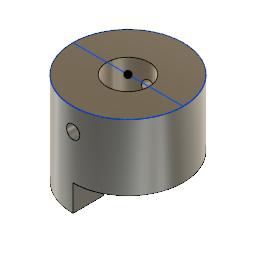
Rotational Link v1 (Autodesk Fusion 360 design; units mm, degrees)
Autodesk Fusion 360 part; units mm, degrees
mesh "Mesh1" [no effect]
sketch "Sketch1" plane through (0, 0, 0) normal (0, 0, 1) x (1, 0, 0)
  spline S0 degree 5 poles (-0.6, 6.1514) (-0.576, 6.0983) (-0.528, 5.9968) (-0.456, 5.8583) (-0.36, 5.7021) (-0.24, 5.5571) (-0.12, 5.4669) (0, 5.436) (0.12, 5.4669) (0.24, 5.5571) (0.36, 5.7021) (0.456, 5.8583) (0.528, 5.9968) (0.576, 6.0983) (0.6, 6.1514) knots 0 0 0 0 0 0 0.1 0.2 0.3 0.4 0.5 0.6 0.7 0.8 0.9 1 1 1 1 1 1
  spline S1 degree 5 poles (-0.6, 6.1514) (-0.576, 6.0983) (-0.528, 5.9968) (-0.456, 5.8583) (-0.36, 5.7021) (-0.24, 5.5571) (-0.12, 5.4669) (0, 5.436) (0.12, 5.4669) (0.24, 5.5571) (0.36, 5.7021) (0.456, 5.8583) (0.528, 5.9968) (0.576, 6.0983) (0.6, 6.1514) knots 0 0 0 0 0 0 0.1 0.2 0.3 0.4 0.5 0.6 0.7 0.8 0.9 1 1 1 1 1 1
  line L0 (0.6, 6.1514) -> (1.3338, 6.0301)
  spline S2 degree 5 poles (-2.4715, 5.6649) (-2.4323, 5.6218) (-2.3553, 5.5401) (-2.244, 5.4307) (-2.1044, 5.3117) (-1.9455, 5.2109) (-1.8035, 5.1622) (-1.6798, 5.1699) (-1.5752, 5.2364) (-1.489, 5.3592) (-1.4197, 5.5342) (-1.3767, 5.7125) (-1.3509, 5.8664) (-1.3367, 5.9778) (-1.3303, 6.0357) knots 0 0 0 0 0 0 0.1 0.2 0.3 0.4 0.5 0.6 0.7 0.8 0.9 1 1 1 1 1 1
  line L1 (-1.3303, 6.0357) -> (-0.5949, 6.1471)
  spline S3 degree 5 poles (-4.1011, 4.6239) (-4.0505, 4.5951) (-3.952, 4.5411) (-3.8124, 4.4715) (-3.6428, 4.4015) (-3.4605, 4.3547) (-3.3104, 4.3523) (-3.1952, 4.3978) (-3.1163, 4.4933) (-3.0722, 4.6368) (-3.0603, 4.8247) (-3.0745, 5.0075) (-3.0976, 5.1618) (-3.1185, 5.2722) (-3.1303, 5.3292) knots 0 0 0 0 0 0 0.1 0.2 0.3 0.4 0.5 0.6 0.7 0.8 0.9 1 1 1 1 1 1
  line L2 (-3.1303, 5.3292) -> (-2.4653, 5.6624)
  spline S4 degree 5 poles (-5.3293, 3.1303) (-5.2722, 3.1185) (-5.1618, 3.0976) (-5.0075, 3.0745) (-4.8247, 3.0603) (-4.6368, 3.0722) (-4.4933, 3.1163) (-4.3978, 3.1952) (-4.3523, 3.3104) (-4.3547, 3.4605) (-4.4015, 3.6428) (-4.4715, 3.8123) (-4.5411, 3.952) (-4.5951, 4.0505) (-4.6239, 4.1011) knots 0 0 0 0 0 0 0.1 0.2 0.3 0.4 0.5 0.6 0.7 0.8 0.9 1 1 1 1 1 1
  line L3 (-4.6239, 4.1011) -> (-4.0944, 4.6234)
  spline S5 degree 5 poles (-6.0357, 1.3302) (-5.9778, 1.3367) (-5.8664, 1.3509) (-5.7125, 1.3766) (-5.5342, 1.4196) (-5.3592, 1.489) (-5.2364, 1.5752) (-5.1699, 1.6798) (-5.1622, 1.8035) (-5.2109, 1.9455) (-5.3117, 2.1044) (-5.4307, 2.244) (-5.5401, 2.3552) (-5.6218, 2.4323) (-5.6649, 2.4715) knots 0 0 0 0 0 0 0.1 0.2 0.3 0.4 0.5 0.6 0.7 0.8 0.9 1 1 1 1 1 1
  line L4 (-5.6649, 2.4715) -> (-5.3228, 3.1319)
  spline S6 degree 5 poles (-6.1514, -0.6) (-6.0983, -0.576) (-5.9968, -0.528) (-5.8583, -0.456) (-5.7021, -0.36) (-5.5571, -0.24) (-5.4669, -0.12) (-5.436, 0) (-5.4669, 0.12) (-5.5571, 0.24) (-5.7021, 0.36) (-5.8583, 0.456) (-5.9968, 0.528) (-6.0983, 0.576) (-6.1514, 0.6) knots 0 0 0 0 0 0 0.1 0.2 0.3 0.4 0.5 0.6 0.7 0.8 0.9 1 1 1 1 1 1
  line L5 (-6.1514, 0.6) -> (-6.0301, 1.3338)
  spline S7 degree 5 poles (-5.6649, -2.4715) (-5.6218, -2.4323) (-5.5401, -2.3553) (-5.4307, -2.244) (-5.3117, -2.1044) (-5.2109, -1.9455) (-5.1622, -1.8035) (-5.1699, -1.6798) (-5.2364, -1.5752) (-5.3592, -1.489) (-5.5342, -1.4197) (-5.7125, -1.3767) (-5.8664, -1.3509) (-5.9778, -1.3367) (-6.0357, -1.3303) knots 0 0 0 0 0 0 0.1 0.2 0.3 0.4 0.5 0.6 0.7 0.8 0.9 1 1 1 1 1 1
  line L6 (-6.0357, -1.3303) -> (-6.1471, -0.5949)
  spline S8 degree 5 poles (-4.6239, -4.1011) (-4.5951, -4.0505) (-4.5411, -3.952) (-4.4715, -3.8124) (-4.4015, -3.6428) (-4.3547, -3.4605) (-4.3523, -3.3104) (-4.3978, -3.1952) (-4.4933, -3.1163) (-4.6368, -3.0722) (-4.8247, -3.0603) (-5.0075, -3.0745) (-5.1618, -3.0976) (-5.2722, -3.1185) (-5.3292, -3.1303) knots 0 0 0 0 0 0 0.1 0.2 0.3 0.4 0.5 0.6 0.7 0.8 0.9 1 1 1 1 1 1
  line L7 (-5.3292, -3.1303) -> (-5.6624, -2.4653)
  spline S9 degree 5 poles (-3.1303, -5.3293) (-3.1185, -5.2722) (-3.0976, -5.1618) (-3.0745, -5.0075) (-3.0603, -4.8247) (-3.0722, -4.6368) (-3.1163, -4.4933) (-3.1952, -4.3978) (-3.3104, -4.3523) (-3.4605, -4.3547) (-3.6428, -4.4015) (-3.8123, -4.4715) (-3.952, -4.5411) (-4.0505, -4.5951) (-4.1011, -4.6239) knots 0 0 0 0 0 0 0.1 0.2 0.3 0.4 0.5 0.6 0.7 0.8 0.9 1 1 1 1 1 1
  line L8 (-4.1011, -4.6239) -> (-4.6234, -4.0944)
  spline S10 degree 5 poles (-1.3302, -6.0357) (-1.3367, -5.9778) (-1.3509, -5.8664) (-1.3766, -5.7125) (-1.4196, -5.5342) (-1.489, -5.3592) (-1.5752, -5.2364) (-1.6798, -5.1699) (-1.8035, -5.1622) (-1.9455, -5.2109) (-2.1044, -5.3117) (-2.244, -5.4307) (-2.3552, -5.5401) (-2.4323, -5.6218) (-2.4715, -5.6649) knots 0 0 0 0 0 0 0.1 0.2 0.3 0.4 0.5 0.6 0.7 0.8 0.9 1 1 1 1 1 1
  line L9 (-2.4715, -5.6649) -> (-3.1319, -5.3228)
  spline S11 degree 5 poles (0.6, -6.1514) (0.576, -6.0983) (0.528, -5.9968) (0.456, -5.8583) (0.36, -5.7021) (0.24, -5.5571) (0.12, -5.4669) (0, -5.436) (-0.12, -5.4669) (-0.24, -5.5571) (-0.36, -5.7021) (-0.456, -5.8583) (-0.528, -5.9968) (-0.576, -6.0983) (-0.6, -6.1514) knots 0 0 0 0 0 0 0.1 0.2 0.3 0.4 0.5 0.6 0.7 0.8 0.9 1 1 1 1 1 1
  line L10 (-0.6, -6.1514) -> (-1.3338, -6.0301)
  spline S12 degree 5 poles (2.4715, -5.6649) (2.4323, -5.6218) (2.3553, -5.5401) (2.244, -5.4307) (2.1044, -5.3117) (1.9455, -5.2109) (1.8035, -5.1622) (1.6798, -5.1699) (1.5752, -5.2364) (1.489, -5.3592) (1.4197, -5.5342) (1.3767, -5.7125) (1.3509, -5.8664) (1.3367, -5.9778) (1.3303, -6.0357) knots 0 0 0 0 0 0 0.1 0.2 0.3 0.4 0.5 0.6 0.7 0.8 0.9 1 1 1 1 1 1
  line L11 (1.3303, -6.0357) -> (0.5949, -6.1471)
  spline S13 degree 5 poles (4.1011, -4.6239) (4.0505, -4.5951) (3.952, -4.5411) (3.8124, -4.4715) (3.6428, -4.4015) (3.4605, -4.3547) (3.3104, -4.3523) (3.1952, -4.3978) (3.1163, -4.4933) (3.0722, -4.6368) (3.0603, -4.8247) (3.0745, -5.0075) (3.0976, -5.1618) (3.1185, -5.2722) (3.1303, -5.3292) knots 0 0 0 0 0 0 0.1 0.2 0.3 0.4 0.5 0.6 0.7 0.8 0.9 1 1 1 1 1 1
  line L12 (3.1303, -5.3292) -> (2.4653, -5.6624)
  spline S14 degree 5 poles (5.3293, -3.1303) (5.2722, -3.1185) (5.1618, -3.0976) (5.0075, -3.0745) (4.8247, -3.0603) (4.6368, -3.0722) (4.4933, -3.1163) (4.3978, -3.1952) (4.3523, -3.3104) (4.3547, -3.4605) (4.4015, -3.6428) (4.4715, -3.8123) (4.5411, -3.952) (4.5951, -4.0505) (4.6239, -4.1011) knots 0 0 0 0 0 0 0.1 0.2 0.3 0.4 0.5 0.6 0.7 0.8 0.9 1 1 1 1 1 1
  line L13 (4.6239, -4.1011) -> (4.0944, -4.6234)
  spline S15 degree 5 poles (6.0357, -1.3302) (5.9778, -1.3367) (5.8664, -1.3509) (5.7125, -1.3766) (5.5342, -1.4196) (5.3592, -1.489) (5.2364, -1.5752) (5.1699, -1.6798) (5.1622, -1.8035) (5.2109, -1.9455) (5.3117, -2.1044) (5.4307, -2.244) (5.5401, -2.3552) (5.6218, -2.4323) (5.6649, -2.4715) knots 0 0 0 0 0 0 0.1 0.2 0.3 0.4 0.5 0.6 0.7 0.8 0.9 1 1 1 1 1 1
  line L14 (5.6649, -2.4715) -> (5.3228, -3.1319)
  spline S16 degree 5 poles (6.1514, 0.6) (6.0983, 0.576) (5.9968, 0.528) (5.8583, 0.456) (5.7021, 0.36) (5.5571, 0.24) (5.4669, 0.12) (5.436, 0) (5.4669, -0.12) (5.5571, -0.24) (5.7021, -0.36) (5.8583, -0.456) (5.9968, -0.528) (6.0983, -0.576) (6.1514, -0.6) knots 0 0 0 0 0 0 0.1 0.2 0.3 0.4 0.5 0.6 0.7 0.8 0.9 1 1 1 1 1 1
  line L15 (6.1514, -0.6) -> (6.0301, -1.3338)
  spline S17 degree 5 poles (5.6649, 2.4715) (5.6218, 2.4323) (5.5401, 2.3553) (5.4307, 2.244) (5.3117, 2.1044) (5.2109, 1.9455) (5.1622, 1.8035) (5.1699, 1.6798) (5.2364, 1.5752) (5.3592, 1.489) (5.5342, 1.4197) (5.7125, 1.3767) (5.8664, 1.3509) (5.9778, 1.3367) (6.0357, 1.3303) knots 0 0 0 0 0 0 0.1 0.2 0.3 0.4 0.5 0.6 0.7 0.8 0.9 1 1 1 1 1 1
  line L16 (6.0357, 1.3303) -> (6.1471, 0.5949)
  spline S18 degree 5 poles (4.6239, 4.1011) (4.5951, 4.0505) (4.5411, 3.952) (4.4715, 3.8124) (4.4015, 3.6428) (4.3547, 3.4605) (4.3523, 3.3104) (4.3978, 3.1952) (4.4933, 3.1163) (4.6368, 3.0722) (4.8247, 3.0603) (5.0075, 3.0745) (5.1618, 3.0976) (5.2722, 3.1185) (5.3292, 3.1303) knots 0 0 0 0 0 0 0.1 0.2 0.3 0.4 0.5 0.6 0.7 0.8 0.9 1 1 1 1 1 1
  line L17 (5.3292, 3.1303) -> (5.6624, 2.4653)
  spline S19 degree 5 poles (3.1303, 5.3293) (3.1185, 5.2722) (3.0976, 5.1618) (3.0745, 5.0075) (3.0603, 4.8247) (3.0722, 4.6368) (3.1163, 4.4933) (3.1952, 4.3978) (3.3104, 4.3523) (3.4605, 4.3547) (3.6428, 4.4015) (3.8123, 4.4715) (3.952, 4.5411) (4.0505, 4.5951) (4.1011, 4.6239) knots 0 0 0 0 0 0 0.1 0.2 0.3 0.4 0.5 0.6 0.7 0.8 0.9 1 1 1 1 1 1
  line L18 (4.1011, 4.6239) -> (4.6234, 4.0944)
  spline S20 degree 5 poles (1.3302, 6.0357) (1.3367, 5.9778) (1.3509, 5.8664) (1.3766, 5.7125) (1.4196, 5.5342) (1.489, 5.3592) (1.5752, 5.2364) (1.6798, 5.1699) (1.8035, 5.1622) (1.9455, 5.2109) (2.1044, 5.3117) (2.244, 5.4307) (2.3552, 5.5401) (2.4323, 5.6218) (2.4715, 5.6649) knots 0 0 0 0 0 0 0.1 0.2 0.3 0.4 0.5 0.6 0.7 0.8 0.9 1 1 1 1 1 1
  line L19 (2.4715, 5.6649) -> (3.1319, 5.3228)
  circle A0 centre (0, 0) radius 12.5
  point P0 (0, 5.4514)
  point P1 (0, 5.4514)
  point P2 (-1.6846, 5.1846)
  point P3 (-3.2043, 4.4103)
  point P4 (-4.4103, 3.2042)
  point P5 (-5.1846, 1.6846)
  point P6 (-5.4514, 0)
  point P7 (-5.1846, -1.6846)
  point P8 (-4.4103, -3.2043)
  point P9 (-3.2042, -4.4103)
  point P10 (-1.6846, -5.1846)
  point P11 (0, -5.4514)
  point P12 (1.6846, -5.1846)
  point P13 (3.2043, -4.4103)
  point P14 (4.4103, -3.2042)
  point P15 (5.1846, -1.6846)
  point P16 (5.4514, 0)
  point P17 (5.1846, 1.6846)
  point P18 (4.4103, 3.2043)
  point P19 (3.2042, 4.4103)
  point P20 (1.6846, 5.1846)
  constraint coincident A0.centre origin
extrude "Extrude1" add sketch "Sketch1" along normal blind 6
sketch "Sketch2" plane through (0, 0, 6) normal (0, 0, 1) x (-1, 0, 0)
  spline S0 degree 5 poles (-1.3308, -6.0305) (-1.3372, -5.9738) (-1.3514, -5.8637) (-1.377, -5.7109) (-1.4199, -5.5336) (-1.489, -5.3592) (-1.5752, -5.2364) (-1.6798, -5.1699) (-1.8035, -5.1622) (-1.9455, -5.2109) (-2.1044, -5.3117) (-2.244, -5.4307) (-2.3552, -5.5401) (-2.4323, -5.6218) (-2.4715, -5.6649) knots 0.001796 0.001796 0.001796 0.001796 0.001796 0.001796 0.1 0.2 0.3 0.4 0.5 0.6 0.7 0.8 0.9 1 1 1 1 1 1
  line L0 (-2.4715, -5.6649) -> (-3.1292, -5.3241)
  spline S1 degree 5 poles (-3.1292, -5.3241) (-3.1177, -5.2682) (-3.0972, -5.1591) (-3.0744, -5.0059) (-3.0604, -4.824) (-3.0722, -4.6368) (-3.1163, -4.4933) (-3.1952, -4.3978) (-3.3104, -4.3523) (-3.4605, -4.3547) (-3.6428, -4.4015) (-3.8123, -4.4715) (-3.952, -4.5411) (-4.0505, -4.5951) (-4.1011, -4.6239) knots 0.001796 0.001796 0.001796 0.001796 0.001796 0.001796 0.1 0.2 0.3 0.4 0.5 0.6 0.7 0.8 0.9 1 1 1 1 1 1
  line L1 (-4.1011, -4.6239) -> (-4.6213, -4.0966)
  spline S2 degree 5 poles (-4.6213, -4.0966) (-4.5931, -4.047) (-4.5399, -3.9495) (-4.4708, -3.8108) (-4.4013, -3.6422) (-4.3547, -3.4605) (-4.3523, -3.3104) (-4.3978, -3.1952) (-4.4933, -3.1163) (-4.6368, -3.0722) (-4.8247, -3.0603) (-5.0075, -3.0745) (-5.1618, -3.0976) (-5.2722, -3.1185) (-5.3292, -3.1303) knots 0.001796 0.001796 0.001796 0.001796 0.001796 0.001796 0.1 0.2 0.3 0.4 0.5 0.6 0.7 0.8 0.9 1 1 1 1 1 1
  line L2 (-5.3292, -3.1303) -> (-5.6611, -2.468)
  spline S3 degree 5 poles (-5.6611, -2.468) (-5.6189, -2.4295) (-5.5381, -2.3533) (-5.4296, -2.2428) (-5.3114, -2.1039) (-5.2109, -1.9455) (-5.1622, -1.8035) (-5.1699, -1.6798) (-5.2364, -1.5752) (-5.3592, -1.489) (-5.5342, -1.4197) (-5.7125, -1.3767) (-5.8664, -1.3509) (-5.9778, -1.3367) (-6.0357, -1.3303) knots 0.001796 0.001796 0.001796 0.001796 0.001796 0.001796 0.1 0.2 0.3 0.4 0.5 0.6 0.7 0.8 0.9 1 1 1 1 1 1
  line L3 (-6.0357, -1.3303) -> (-6.1466, -0.5979)
  spline S4 degree 5 poles (-6.1466, -0.5979) (-6.0947, -0.5743) (-5.9943, -0.5267) (-5.8569, -0.4551) (-5.7015, -0.3596) (-5.5571, -0.24) (-5.4669, -0.12) (-5.436, 0) (-5.4669, 0.12) (-5.5571, 0.24) (-5.7021, 0.36) (-5.8583, 0.456) (-5.9968, 0.528) (-6.0983, 0.576) (-6.1514, 0.6) knots 0.001796 0.001796 0.001796 0.001796 0.001796 0.001796 0.1 0.2 0.3 0.4 0.5 0.6 0.7 0.8 0.9 1 1 1 1 1 1
  line L4 (-6.1514, 0.6) -> (-6.0305, 1.3308)
  spline S5 degree 5 poles (-6.0305, 1.3308) (-5.9738, 1.3372) (-5.8637, 1.3514) (-5.7109, 1.377) (-5.5336, 1.4199) (-5.3592, 1.489) (-5.2364, 1.5752) (-5.1699, 1.6798) (-5.1622, 1.8035) (-5.2109, 1.9455) (-5.3117, 2.1044) (-5.4307, 2.244) (-5.5401, 2.3552) (-5.6218, 2.4323) (-5.6649, 2.4715) knots 0.001796 0.001796 0.001796 0.001796 0.001796 0.001796 0.1 0.2 0.3 0.4 0.5 0.6 0.7 0.8 0.9 1 1 1 1 1 1
  line L5 (-5.6649, 2.4715) -> (-5.3241, 3.1292)
  spline S6 degree 5 poles (-5.3241, 3.1292) (-5.2682, 3.1177) (-5.1591, 3.0972) (-5.0059, 3.0744) (-4.824, 3.0604) (-4.6368, 3.0722) (-4.4933, 3.1163) (-4.3978, 3.1952) (-4.3523, 3.3104) (-4.3547, 3.4605) (-4.4015, 3.6428) (-4.4715, 3.8123) (-4.5411, 3.952) (-4.5951, 4.0505) (-4.6239, 4.1011) knots 0.001796 0.001796 0.001796 0.001796 0.001796 0.001796 0.1 0.2 0.3 0.4 0.5 0.6 0.7 0.8 0.9 1 1 1 1 1 1
  line L6 (-4.6239, 4.1011) -> (-4.0966, 4.6213)
  spline S7 degree 5 poles (-4.0966, 4.6213) (-4.047, 4.5931) (-3.9495, 4.5399) (-3.8108, 4.4708) (-3.6422, 4.4013) (-3.4605, 4.3547) (-3.3104, 4.3523) (-3.1952, 4.3978) (-3.1163, 4.4933) (-3.0722, 4.6368) (-3.0603, 4.8247) (-3.0745, 5.0075) (-3.0976, 5.1618) (-3.1185, 5.2722) (-3.1303, 5.3292) knots 0.001796 0.001796 0.001796 0.001796 0.001796 0.001796 0.1 0.2 0.3 0.4 0.5 0.6 0.7 0.8 0.9 1 1 1 1 1 1
  line L7 (-3.1303, 5.3292) -> (-2.468, 5.6611)
  spline S8 degree 5 poles (-2.468, 5.6611) (-2.4295, 5.6189) (-2.3533, 5.5381) (-2.2428, 5.4296) (-2.1039, 5.3114) (-1.9455, 5.2109) (-1.8035, 5.1622) (-1.6798, 5.1699) (-1.5752, 5.2364) (-1.489, 5.3592) (-1.4197, 5.5342) (-1.3767, 5.7125) (-1.3509, 5.8664) (-1.3367, 5.9778) (-1.3303, 6.0357) knots 0.001796 0.001796 0.001796 0.001796 0.001796 0.001796 0.1 0.2 0.3 0.4 0.5 0.6 0.7 0.8 0.9 1 1 1 1 1 1
  line L8 (-1.3303, 6.0357) -> (-0.5979, 6.1466)
  spline S9 degree 5 poles (-0.5979, 6.1466) (-0.5743, 6.0947) (-0.5267, 5.9943) (-0.4551, 5.8569) (-0.3596, 5.7015) (-0.24, 5.5571) (-0.12, 5.4669) (0, 5.436) (0.12, 5.4669) (0.24, 5.5571) (0.36, 5.7021) (0.456, 5.8583) (0.528, 5.9968) (0.576, 6.0983) (0.6, 6.1514) knots 0.001796 0.001796 0.001796 0.001796 0.001796 0.001796 0.1 0.2 0.3 0.4 0.5 0.6 0.7 0.8 0.9 1 1 1 1 1 1
  line L9 (0.6, 6.1514) -> (1.3308, 6.0305)
  spline S10 degree 5 poles (1.3308, 6.0305) (1.3372, 5.9738) (1.3514, 5.8637) (1.377, 5.7109) (1.4199, 5.5336) (1.489, 5.3592) (1.5752, 5.2364) (1.6798, 5.1699) (1.8035, 5.1622) (1.9455, 5.2109) (2.1044, 5.3117) (2.244, 5.4307) (2.3552, 5.5401) (2.4323, 5.6218) (2.4715, 5.6649) knots 0.001796 0.001796 0.001796 0.001796 0.001796 0.001796 0.1 0.2 0.3 0.4 0.5 0.6 0.7 0.8 0.9 1 1 1 1 1 1
  line L10 (2.4715, 5.6649) -> (3.1292, 5.3241)
  spline S11 degree 5 poles (3.1292, 5.3241) (3.1177, 5.2682) (3.0972, 5.1591) (3.0744, 5.0059) (3.0604, 4.824) (3.0722, 4.6368) (3.1163, 4.4933) (3.1952, 4.3978) (3.3104, 4.3523) (3.4605, 4.3547) (3.6428, 4.4015) (3.8123, 4.4715) (3.952, 4.5411) (4.0505, 4.5951) (4.1011, 4.6239) knots 0.001796 0.001796 0.001796 0.001796 0.001796 0.001796 0.1 0.2 0.3 0.4 0.5 0.6 0.7 0.8 0.9 1 1 1 1 1 1
  line L11 (4.1011, 4.6239) -> (4.6213, 4.0966)
  spline S12 degree 5 poles (4.6213, 4.0966) (4.5931, 4.047) (4.5399, 3.9495) (4.4708, 3.8108) (4.4013, 3.6422) (4.3547, 3.4605) (4.3523, 3.3104) (4.3978, 3.1952) (4.4933, 3.1163) (4.6368, 3.0722) (4.8247, 3.0603) (5.0075, 3.0745) (5.1618, 3.0976) (5.2722, 3.1185) (5.3292, 3.1303) knots 0.001796 0.001796 0.001796 0.001796 0.001796 0.001796 0.1 0.2 0.3 0.4 0.5 0.6 0.7 0.8 0.9 1 1 1 1 1 1
  line L12 (5.3292, 3.1303) -> (5.6611, 2.468)
  spline S13 degree 5 poles (5.6611, 2.468) (5.6189, 2.4295) (5.5381, 2.3533) (5.4296, 2.2428) (5.3114, 2.1039) (5.2109, 1.9455) (5.1622, 1.8035) (5.1699, 1.6798) (5.2364, 1.5752) (5.3592, 1.489) (5.5342, 1.4197) (5.7125, 1.3767) (5.8664, 1.3509) (5.9778, 1.3367) (6.0357, 1.3303) knots 0.001796 0.001796 0.001796 0.001796 0.001796 0.001796 0.1 0.2 0.3 0.4 0.5 0.6 0.7 0.8 0.9 1 1 1 1 1 1
  line L13 (6.0357, 1.3303) -> (6.1466, 0.5979)
  spline S14 degree 5 poles (6.1466, 0.5979) (6.0947, 0.5743) (5.9943, 0.5267) (5.8569, 0.4551) (5.7015, 0.3596) (5.5571, 0.24) (5.4669, 0.12) (5.436, 0) (5.4669, -0.12) (5.5571, -0.24) (5.7021, -0.36) (5.8583, -0.456) (5.9968, -0.528) (6.0983, -0.576) (6.1514, -0.6) knots 0.001796 0.001796 0.001796 0.001796 0.001796 0.001796 0.1 0.2 0.3 0.4 0.5 0.6 0.7 0.8 0.9 1 1 1 1 1 1
  line L14 (6.1514, -0.6) -> (6.0305, -1.3308)
  spline S15 degree 5 poles (6.0305, -1.3308) (5.9738, -1.3372) (5.8637, -1.3514) (5.7109, -1.377) (5.5336, -1.4199) (5.3592, -1.489) (5.2364, -1.5752) (5.1699, -1.6798) (5.1622, -1.8035) (5.2109, -1.9455) (5.3117, -2.1044) (5.4307, -2.244) (5.5401, -2.3552) (5.6218, -2.4323) (5.6649, -2.4715) knots 0.001796 0.001796 0.001796 0.001796 0.001796 0.001796 0.1 0.2 0.3 0.4 0.5 0.6 0.7 0.8 0.9 1 1 1 1 1 1
  line L15 (5.6649, -2.4715) -> (5.3241, -3.1292)
  spline S16 degree 5 poles (5.3241, -3.1292) (5.2682, -3.1177) (5.1591, -3.0972) (5.0059, -3.0744) (4.824, -3.0604) (4.6368, -3.0722) (4.4933, -3.1163) (4.3978, -3.1952) (4.3523, -3.3104) (4.3547, -3.4605) (4.4015, -3.6428) (4.4715, -3.8123) (4.5411, -3.952) (4.5951, -4.0505) (4.6239, -4.1011) knots 0.001796 0.001796 0.001796 0.001796 0.001796 0.001796 0.1 0.2 0.3 0.4 0.5 0.6 0.7 0.8 0.9 1 1 1 1 1 1
  line L16 (4.6239, -4.1011) -> (4.0966, -4.6213)
  spline S17 degree 5 poles (4.0966, -4.6213) (4.047, -4.5931) (3.9495, -4.5399) (3.8108, -4.4708) (3.6422, -4.4013) (3.4605, -4.3547) (3.3104, -4.3523) (3.1952, -4.3978) (3.1163, -4.4933) (3.0722, -4.6368) (3.0603, -4.8247) (3.0745, -5.0075) (3.0976, -5.1618) (3.1185, -5.2722) (3.1303, -5.3292) knots 0.001796 0.001796 0.001796 0.001796 0.001796 0.001796 0.1 0.2 0.3 0.4 0.5 0.6 0.7 0.8 0.9 1 1 1 1 1 1
  line L17 (3.1303, -5.3292) -> (2.468, -5.6611)
  spline S18 degree 5 poles (2.468, -5.6611) (2.4295, -5.6189) (2.3533, -5.5381) (2.2428, -5.4296) (2.1039, -5.3114) (1.9455, -5.2109) (1.8035, -5.1622) (1.6798, -5.1699) (1.5752, -5.2364) (1.489, -5.3592) (1.4197, -5.5342) (1.3767, -5.7125) (1.3509, -5.8664) (1.3367, -5.9778) (1.3303, -6.0357) knots 0.001796 0.001796 0.001796 0.001796 0.001796 0.001796 0.1 0.2 0.3 0.4 0.5 0.6 0.7 0.8 0.9 1 1 1 1 1 1
  line L18 (1.3303, -6.0357) -> (0.5979, -6.1466)
  spline S19 degree 5 poles (0.5979, -6.1466) (0.5743, -6.0947) (0.5267, -5.9943) (0.4551, -5.8569) (0.3596, -5.7015) (0.24, -5.5571) (0.12, -5.4669) (0, -5.436) (-0.12, -5.4669) (-0.24, -5.5571) (-0.36, -5.7021) (-0.456, -5.8583) (-0.528, -5.9968) (-0.576, -6.0983) (-0.6, -6.1514) knots 0.001796 0.001796 0.001796 0.001796 0.001796 0.001796 0.1 0.2 0.3 0.4 0.5 0.6 0.7 0.8 0.9 1 1 1 1 1 1
  line L19 (-0.6, -6.1514) -> (-1.3308, -6.0305)
  circle A0 centre (0, 0) radius 12.5
  circle A1 centre (0, 0) radius 7.75
  circle A2 centre (0, 0) radius 12.5
  dimension "d5" = 15.5
  constraint concentric A0 A1
  constraint concentric A0 A2
  measures "d5" diameter of A1
extrude "Extrude2" add sketch "Sketch2" along normal blind 2 contours A0 A2
sketch "Sketch3" plane through (0, 0, 8) normal (0, 0, 1) x (-1, 0, 0)
  circle A0 centre (0, 0) radius 7.75
  circle A1 centre (0, 0) radius 12.5
  circle A2 centre (0, 0) radius 12.5
  constraint coincident A0.centre A1.centre
extrude "Extrude3" add sketch "Sketch3" along normal blind 3 contours A0 | A1 A2
sketch "Sketch4" plane through (0, 0, 11) normal (0, 0, 1) x (-1, 0, 0)
  circle A0 centre (0, 0) radius 12.5
extrude "Extrude4" add sketch "Sketch4" along normal blind 10
sketch "Sketch5" plane through (0, 0, 21) normal (0, 0, 1) x (-1, 0, 0)
  circle A0 centre (0, 0) radius 12.5
  circle A1 centre (0, 0) radius 4.775
  dimension "d12" = 9.55
  constraint concentric A0 A1
  measures "d12" diameter of A1
extrude "Extrude5" cut sketch "Sketch5" against normal blind 10 contours A1
sketch "Sketch6" plane through (0, 0, 0) normal (0, 1, 0) x (1, 0, 0)
  line L0 (0, -21) -> (0, -16)
  circle A0 centre (0, -16) radius 1.5
  dimension "d15" = 5
  dimension "d16" = 3
  constraint vertical L0
  constraint coincident L0.end A0.centre
  measures "d15" distance of L0.start L0.end
  measures "d16" diameter of A0
extrude "Extrude6" cut sketch "Sketch6" against normal through all and the other way through all
sketch "Sketch7" plane through (0, 0, 21) normal (0, 0, 1) x (-1, 0, 0)
  circle A0 centre (0, 0) radius 4.775
  circle A1 centre (0, 0) radius 12.5
  circle A2 centre (0, 0) radius 12.5
  line L0 (12.5, 0) -> (-12.5, 0)
  constraint coincident A0.centre A1.centre
  constraint coincident A2 L0.start
  constraint coincident A2 L0.end
  constraint horizontal L0
sketch "Sketch8" plane through (0, 0, 0) normal (0, 0, -1) x (1, 0, 0)
  spline S0 degree 5 poles (1.3308, -6.0305) (1.3372, -5.9738) (1.3514, -5.8637) (1.377, -5.7109) (1.4199, -5.5336) (1.489, -5.3592) (1.5752, -5.2364) (1.6798, -5.1699) (1.8035, -5.1622) (1.9455, -5.2109) (2.1044, -5.3117) (2.244, -5.4307) (2.3552, -5.5401) (2.4323, -5.6218) (2.4715, -5.6649) knots 0.001796 0.001796 0.001796 0.001796 0.001796 0.001796 0.1 0.2 0.3 0.4 0.5 0.6 0.7 0.8 0.9 1 1 1 1 1 1
  line L0 (1.3308, -6.0305) -> (0.6, -6.1514)
  spline S1 degree 5 poles (-0.5979, -6.1466) (-0.5743, -6.0947) (-0.5267, -5.9943) (-0.4551, -5.8569) (-0.3596, -5.7015) (-0.24, -5.5571) (-0.12, -5.4669) (0, -5.436) (0.12, -5.4669) (0.24, -5.5571) (0.36, -5.7021) (0.456, -5.8583) (0.528, -5.9968) (0.576, -6.0983) (0.6, -6.1514) knots 0.001796 0.001796 0.001796 0.001796 0.001796 0.001796 0.1 0.2 0.3 0.4 0.5 0.6 0.7 0.8 0.9 1 1 1 1 1 1
  line L1 (-0.5979, -6.1466) -> (-1.3303, -6.0357)
  spline S2 degree 5 poles (-2.468, -5.6611) (-2.4295, -5.6189) (-2.3533, -5.5381) (-2.2428, -5.4296) (-2.1039, -5.3114) (-1.9455, -5.2109) (-1.8035, -5.1622) (-1.6798, -5.1699) (-1.5752, -5.2364) (-1.489, -5.3592) (-1.4197, -5.5342) (-1.3767, -5.7125) (-1.3509, -5.8664) (-1.3367, -5.9778) (-1.3303, -6.0357) knots 0.001796 0.001796 0.001796 0.001796 0.001796 0.001796 0.1 0.2 0.3 0.4 0.5 0.6 0.7 0.8 0.9 1 1 1 1 1 1
  line L2 (-2.468, -5.6611) -> (-3.1303, -5.3292)
  spline S3 degree 5 poles (-4.0966, -4.6213) (-4.047, -4.5931) (-3.9495, -4.5399) (-3.8108, -4.4708) (-3.6422, -4.4013) (-3.4605, -4.3547) (-3.3104, -4.3523) (-3.1952, -4.3978) (-3.1163, -4.4933) (-3.0722, -4.6368) (-3.0603, -4.8247) (-3.0745, -5.0075) (-3.0976, -5.1618) (-3.1185, -5.2722) (-3.1303, -5.3292) knots 0.001796 0.001796 0.001796 0.001796 0.001796 0.001796 0.1 0.2 0.3 0.4 0.5 0.6 0.7 0.8 0.9 1 1 1 1 1 1
  line L3 (-4.0966, -4.6213) -> (-4.6239, -4.1011)
  spline S4 degree 5 poles (-5.3241, -3.1292) (-5.2682, -3.1177) (-5.1591, -3.0972) (-5.0059, -3.0744) (-4.824, -3.0604) (-4.6368, -3.0722) (-4.4933, -3.1163) (-4.3978, -3.1952) (-4.3523, -3.3104) (-4.3547, -3.4605) (-4.4015, -3.6428) (-4.4715, -3.8123) (-4.5411, -3.952) (-4.5951, -4.0505) (-4.6239, -4.1011) knots 0.001796 0.001796 0.001796 0.001796 0.001796 0.001796 0.1 0.2 0.3 0.4 0.5 0.6 0.7 0.8 0.9 1 1 1 1 1 1
  line L4 (-5.3241, -3.1292) -> (-5.6649, -2.4715)
  spline S5 degree 5 poles (-6.0305, -1.3308) (-5.9738, -1.3372) (-5.8637, -1.3514) (-5.7109, -1.377) (-5.5336, -1.4199) (-5.3592, -1.489) (-5.2364, -1.5752) (-5.1699, -1.6798) (-5.1622, -1.8035) (-5.2109, -1.9455) (-5.3117, -2.1044) (-5.4307, -2.244) (-5.5401, -2.3552) (-5.6218, -2.4323) (-5.6649, -2.4715) knots 0.001796 0.001796 0.001796 0.001796 0.001796 0.001796 0.1 0.2 0.3 0.4 0.5 0.6 0.7 0.8 0.9 1 1 1 1 1 1
  line L5 (-6.0305, -1.3308) -> (-6.1514, -0.6)
  spline S6 degree 5 poles (-6.1466, 0.5979) (-6.0947, 0.5743) (-5.9943, 0.5267) (-5.8569, 0.4551) (-5.7015, 0.3596) (-5.5571, 0.24) (-5.4669, 0.12) (-5.436, 0) (-5.4669, -0.12) (-5.5571, -0.24) (-5.7021, -0.36) (-5.8583, -0.456) (-5.9968, -0.528) (-6.0983, -0.576) (-6.1514, -0.6) knots 0.001796 0.001796 0.001796 0.001796 0.001796 0.001796 0.1 0.2 0.3 0.4 0.5 0.6 0.7 0.8 0.9 1 1 1 1 1 1
  line L6 (-6.1466, 0.5979) -> (-6.0357, 1.3303)
  spline S7 degree 5 poles (-5.6611, 2.468) (-5.6189, 2.4295) (-5.5381, 2.3533) (-5.4296, 2.2428) (-5.3114, 2.1039) (-5.2109, 1.9455) (-5.1622, 1.8035) (-5.1699, 1.6798) (-5.2364, 1.5752) (-5.3592, 1.489) (-5.5342, 1.4197) (-5.7125, 1.3767) (-5.8664, 1.3509) (-5.9778, 1.3367) (-6.0357, 1.3303) knots 0.001796 0.001796 0.001796 0.001796 0.001796 0.001796 0.1 0.2 0.3 0.4 0.5 0.6 0.7 0.8 0.9 1 1 1 1 1 1
  line L7 (-5.6611, 2.468) -> (-5.3292, 3.1303)
  spline S8 degree 5 poles (-4.6213, 4.0966) (-4.5931, 4.047) (-4.5399, 3.9495) (-4.4708, 3.8108) (-4.4013, 3.6422) (-4.3547, 3.4605) (-4.3523, 3.3104) (-4.3978, 3.1952) (-4.4933, 3.1163) (-4.6368, 3.0722) (-4.8247, 3.0603) (-5.0075, 3.0745) (-5.1618, 3.0976) (-5.2722, 3.1185) (-5.3292, 3.1303) knots 0.001796 0.001796 0.001796 0.001796 0.001796 0.001796 0.1 0.2 0.3 0.4 0.5 0.6 0.7 0.8 0.9 1 1 1 1 1 1
  line L8 (-4.6213, 4.0966) -> (-4.1011, 4.6239)
  spline S9 degree 5 poles (-3.1292, 5.3241) (-3.1177, 5.2682) (-3.0972, 5.1591) (-3.0744, 5.0059) (-3.0604, 4.824) (-3.0722, 4.6368) (-3.1163, 4.4933) (-3.1952, 4.3978) (-3.3104, 4.3523) (-3.4605, 4.3547) (-3.6428, 4.4015) (-3.8123, 4.4715) (-3.952, 4.5411) (-4.0505, 4.5951) (-4.1011, 4.6239) knots 0.001796 0.001796 0.001796 0.001796 0.001796 0.001796 0.1 0.2 0.3 0.4 0.5 0.6 0.7 0.8 0.9 1 1 1 1 1 1
  line L9 (-3.1292, 5.3241) -> (-2.4715, 5.6649)
  spline S10 degree 5 poles (-1.3308, 6.0305) (-1.3372, 5.9738) (-1.3514, 5.8637) (-1.377, 5.7109) (-1.4199, 5.5336) (-1.489, 5.3592) (-1.5752, 5.2364) (-1.6798, 5.1699) (-1.8035, 5.1622) (-1.9455, 5.2109) (-2.1044, 5.3117) (-2.244, 5.4307) (-2.3552, 5.5401) (-2.4323, 5.6218) (-2.4715, 5.6649) knots 0.001796 0.001796 0.001796 0.001796 0.001796 0.001796 0.1 0.2 0.3 0.4 0.5 0.6 0.7 0.8 0.9 1 1 1 1 1 1
  line L10 (-1.3308, 6.0305) -> (-0.6, 6.1514)
  spline S11 degree 5 poles (0.5979, 6.1466) (0.5743, 6.0947) (0.5267, 5.9943) (0.4551, 5.8569) (0.3596, 5.7015) (0.24, 5.5571) (0.12, 5.4669) (0, 5.436) (-0.12, 5.4669) (-0.24, 5.5571) (-0.36, 5.7021) (-0.456, 5.8583) (-0.528, 5.9968) (-0.576, 6.0983) (-0.6, 6.1514) knots 0.001796 0.001796 0.001796 0.001796 0.001796 0.001796 0.1 0.2 0.3 0.4 0.5 0.6 0.7 0.8 0.9 1 1 1 1 1 1
  line L11 (0.5979, 6.1466) -> (1.3303, 6.0357)
  spline S12 degree 5 poles (2.468, 5.6611) (2.4295, 5.6189) (2.3533, 5.5381) (2.2428, 5.4296) (2.1039, 5.3114) (1.9455, 5.2109) (1.8035, 5.1622) (1.6798, 5.1699) (1.5752, 5.2364) (1.489, 5.3592) (1.4197, 5.5342) (1.3767, 5.7125) (1.3509, 5.8664) (1.3367, 5.9778) (1.3303, 6.0357) knots 0.001796 0.001796 0.001796 0.001796 0.001796 0.001796 0.1 0.2 0.3 0.4 0.5 0.6 0.7 0.8 0.9 1 1 1 1 1 1
  line L12 (2.468, 5.6611) -> (3.1303, 5.3292)
  spline S13 degree 5 poles (4.0966, 4.6213) (4.047, 4.5931) (3.9495, 4.5399) (3.8108, 4.4708) (3.6422, 4.4013) (3.4605, 4.3547) (3.3104, 4.3523) (3.1952, 4.3978) (3.1163, 4.4933) (3.0722, 4.6368) (3.0603, 4.8247) (3.0745, 5.0075) (3.0976, 5.1618) (3.1185, 5.2722) (3.1303, 5.3292) knots 0.001796 0.001796 0.001796 0.001796 0.001796 0.001796 0.1 0.2 0.3 0.4 0.5 0.6 0.7 0.8 0.9 1 1 1 1 1 1
  line L13 (4.0966, 4.6213) -> (4.6239, 4.1011)
  spline S14 degree 5 poles (5.3241, 3.1292) (5.2682, 3.1177) (5.1591, 3.0972) (5.0059, 3.0744) (4.824, 3.0604) (4.6368, 3.0722) (4.4933, 3.1163) (4.3978, 3.1952) (4.3523, 3.3104) (4.3547, 3.4605) (4.4015, 3.6428) (4.4715, 3.8123) (4.5411, 3.952) (4.5951, 4.0505) (4.6239, 4.1011) knots 0.001796 0.001796 0.001796 0.001796 0.001796 0.001796 0.1 0.2 0.3 0.4 0.5 0.6 0.7 0.8 0.9 1 1 1 1 1 1
  line L14 (5.3241, 3.1292) -> (5.6649, 2.4715)
  spline S15 degree 5 poles (6.0305, 1.3308) (5.9738, 1.3372) (5.8637, 1.3514) (5.7109, 1.377) (5.5336, 1.4199) (5.3592, 1.489) (5.2364, 1.5752) (5.1699, 1.6798) (5.1622, 1.8035) (5.2109, 1.9455) (5.3117, 2.1044) (5.4307, 2.244) (5.5401, 2.3552) (5.6218, 2.4323) (5.6649, 2.4715) knots 0.001796 0.001796 0.001796 0.001796 0.001796 0.001796 0.1 0.2 0.3 0.4 0.5 0.6 0.7 0.8 0.9 1 1 1 1 1 1
  line L15 (6.0305, 1.3308) -> (6.1514, 0.6)
  spline S16 degree 5 poles (6.1466, -0.5979) (6.0947, -0.5743) (5.9943, -0.5267) (5.8569, -0.4551) (5.7015, -0.3596) (5.5571, -0.24) (5.4669, -0.12) (5.436, 0) (5.4669, 0.12) (5.5571, 0.24) (5.7021, 0.36) (5.8583, 0.456) (5.9968, 0.528) (6.0983, 0.576) (6.1514, 0.6) knots 0.001796 0.001796 0.001796 0.001796 0.001796 0.001796 0.1 0.2 0.3 0.4 0.5 0.6 0.7 0.8 0.9 1 1 1 1 1 1
  line L16 (6.1466, -0.5979) -> (6.0357, -1.3303)
  spline S17 degree 5 poles (5.6611, -2.468) (5.6189, -2.4295) (5.5381, -2.3533) (5.4296, -2.2428) (5.3114, -2.1039) (5.2109, -1.9455) (5.1622, -1.8035) (5.1699, -1.6798) (5.2364, -1.5752) (5.3592, -1.489) (5.5342, -1.4197) (5.7125, -1.3767) (5.8664, -1.3509) (5.9778, -1.3367) (6.0357, -1.3303) knots 0.001796 0.001796 0.001796 0.001796 0.001796 0.001796 0.1 0.2 0.3 0.4 0.5 0.6 0.7 0.8 0.9 1 1 1 1 1 1
  line L17 (5.6611, -2.468) -> (5.3292, -3.1303)
  spline S18 degree 5 poles (4.6213, -4.0966) (4.5931, -4.047) (4.5399, -3.9495) (4.4708, -3.8108) (4.4013, -3.6422) (4.3547, -3.4605) (4.3523, -3.3104) (4.3978, -3.1952) (4.4933, -3.1163) (4.6368, -3.0722) (4.8247, -3.0603) (5.0075, -3.0745) (5.1618, -3.0976) (5.2722, -3.1185) (5.3292, -3.1303) knots 0.001796 0.001796 0.001796 0.001796 0.001796 0.001796 0.1 0.2 0.3 0.4 0.5 0.6 0.7 0.8 0.9 1 1 1 1 1 1
  line L18 (4.6213, -4.0966) -> (4.1011, -4.6239)
  spline S19 degree 5 poles (3.1292, -5.3241) (3.1177, -5.2682) (3.0972, -5.1591) (3.0744, -5.0059) (3.0604, -4.824) (3.0722, -4.6368) (3.1163, -4.4933) (3.1952, -4.3978) (3.3104, -4.3523) (3.4605, -4.3547) (3.6428, -4.4015) (3.8123, -4.4715) (3.952, -4.5411) (4.0505, -4.5951) (4.1011, -4.6239) knots 0.001796 0.001796 0.001796 0.001796 0.001796 0.001796 0.1 0.2 0.3 0.4 0.5 0.6 0.7 0.8 0.9 1 1 1 1 1 1
  line L19 (3.1292, -5.3241) -> (2.4715, -5.6649)
  circle A0 centre (0, 0) radius 12.5
  circle A1 centre (0, 0) radius 12.5
  line L20 (-12.4999, 0.0568) -> (0, 0)
  line L21 (0, 0) -> (-0.0568, -12.4999)
  line L22 (0, 0) -> (12.4999, -0.0568)
  line L23 (0, 0) -> (0.0568, 12.4999)
  constraint coincident A0.centre A1.centre
  constraint coincident A1 L20.start
  constraint coincident A1 L21.end
  constraint perpendicular L20 L21
  constraint coincident A1 L22.end
  constraint perpendicular L21 L22
  constraint coincident A0 L23.end
  constraint perpendicular L22 L23
extrude "Extrude7" cut sketch "Sketch8" against normal blind 6 contours S0 L0 S1 S16 L16 S17 L17 S18 L18 S19 L19 A0 A1 L21 L22 | S1 L1 S2 L2 S3 L3 S4 L4 S5 L5 S6 A0 A1 L20 L21 | S11 L11 S12 L12 S13 L13 S14 L14 S15 L15 S16 A0 A1 L22 L23
